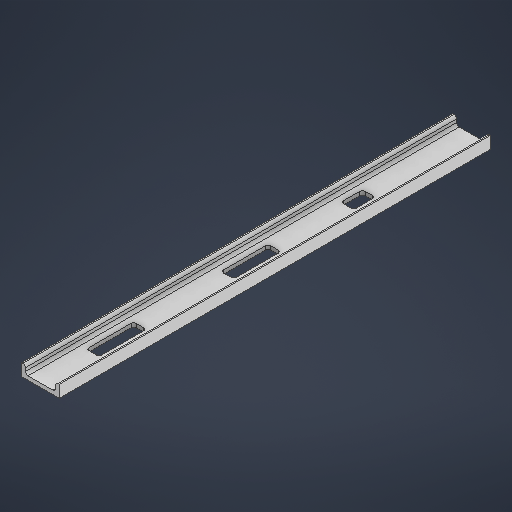
# Autodesk Inventor part: 2 часть направляшки 35
Saved by Autodesk Inventor 2025 (Build 290162000, 162)
## iProperties
Created: 2024-11-23
Part Number: 2 часть направляшки 35
Material: Типовые
Document SubType Name: Modeling
Designer: Phantom
Density: 1 g/cm^3
Appearance: По умолчанию
Author: Phantom
Autodesk Inventor part; units mm, degrees
ref_plane "YZ Plane" through (0, 0, 0) normal (1, 0, 0) x (0, 1, 0)
ref_plane "XZ Plane" through (0, 0, 0) normal (0, 1, 0) x (-1, 0, 0)
ref_plane "XY Plane" through (0, 0, 0) normal (0, 0, 1) x (1, 0, 0)
sketch "Эскиз1" plane through (0, 0, 0) normal (0, 0, 1) x (1, 0, 0)
  line L0 (0, 0) -> (34.5, 0)
  line L1 (34.5, 0) -> (34.5, 9.5)
  line L2 (34.5, 9.5) -> (0, 9.5)
  line L3 (0, 9.5) -> (0, 0)
  line L4 (3, 9.5) -> (3, 0)
  line L5 (31.5, 9.5) -> (31.5, 0)
  line L6 (3, 3) -> (31.5, 3)
  dimension "d0" = 34.5
  dimension "d1" = 9.5
  dimension "d2" = 3
  dimension "d3" = 3
  dimension "d4" = 3
  constraints: 14 end point, 6 point on line, 4 perpendicular, 2 parallel, 1 horizontal
  measures "d0" distance of L2.end L1.end
  measures "d1" distance of L1.end L0.end
  measures "d2" distance between parallel lines of L3 L4
  measures "d3" distance between parallel lines of L5 L1
  measures "d4" distance between parallel lines of L0 L6
extrude "Выдавливание1" add sketch "Эскиз1" along normal blind 388 contours L3 L2 L4 L0 | L4 L6 L5 L0 | L5 L2 L1 L0
sketch "Эскиз2" plane through (0, 0, 0) normal (0, -1, 0) x (1, 0, 0)
  line L0 (0, 0) -> (34.5, 0) projected
  line L1 (34.5, 0) -> (34.5, 388) projected
  line L2 (0, 388) -> (34.5, 388) projected
  line L3 (0, 0) -> (0, 388) projected
  line L4 (17.25, 388) -> (17.25, 0)
  line L5 (22.25, 310) -> (12.25, 310)
  line L6 (12.25, 310) -> (12.25, 347)
  line L7 (12.25, 347) -> (22.25, 347)
  line L8 (22.25, 347) -> (22.25, 310)
  line L9 (22.25, 310) -> (12.25, 347) construction
  line L10 (12.25, 310) -> (22.25, 347) construction
  line L11 (12.25, 204.5) -> (22.25, 204.5)
  line L12 (22.25, 204.5) -> (22.25, 241.5)
  line L13 (22.25, 241.5) -> (12.25, 241.5)
  line L14 (12.25, 241.5) -> (12.25, 204.5)
  line L15 (12.25, 204.5) -> (22.25, 241.5) construction
  line L16 (22.25, 204.5) -> (12.25, 241.5) construction
  line L17 (22.25, 130.5) -> (12.25, 130.5)
  line L18 (12.25, 130.5) -> (12.25, 147.5)
  line L19 (12.25, 147.5) -> (22.25, 147.5)
  line L20 (22.25, 147.5) -> (22.25, 130.5)
  line L21 (22.25, 130.5) -> (12.25, 147.5) construction
  line L22 (12.25, 130.5) -> (22.25, 147.5) construction
  point P0 (17.25, 328.5)
  point P1 (17.25, 223)
  point P2 (17.25, 139)
  dimension "d8" = 10
  dimension "d9" = 37
  dimension "d10" = 41
  dimension "d11" = 10
  dimension "d12" = 37
  dimension "d13" = 68.5
  dimension "d14" = 10
  dimension "d15" = 17
  dimension "d16" = 57
  constraints: 38 end point, 8 midpoint, 6 parallel, 3 horizontal, 3 perpendicular, 3 point on line
  measures "d8" distance of L6.end L7.end
  measures "d9" distance of L5.end L6.end
  measures "d10" distance between parallel lines of L7 L2
  measures "d11" distance of L13.end L12.end
  measures "d12" distance of L12.end L11.end
  measures "d13" distance between parallel lines of L13 L5
  measures "d14" distance of L18.end L19.end
  measures "d15" distance of L17.end L18.end
  measures "d16" distance between parallel lines of L19 L11
extrude "Выдавливание2" cut sketch "Эскиз2" against normal blind 295 contours L17 L18 L19 L4 | L4 L19 L20 L17 | L7 L8 L5 L4 | L4 L5 L6 L7 | L11 L14 L13 L4 | L4 L13 L12 L11
fillet "Сопряжение2" radius 2 12 edges at (12.25, 1.5, 241.5) (12.25, 1.5, 204.5) (22.25, 1.5, 204.5) (22.25, 1.5, 241.5) (22.25, 1.5, 147.5) (22.25, 1.5, 130.5) (12.25, 1.5, 147.5) (12.25, 1.5, 130.5) (12.25, 1.5, 310) (12.25, 1.5, 347) (22.25, 1.5, 347) (22.25, 1.5, 310)
sketch "Эскиз3" plane through (0, 0, 388) normal (0, 0, 1) x (1, 0, 0)
  line L0 (3, 3) -> (3, 9.5) projected
  line L1 (3, 9.5) -> (5.5, 9.5)
  line L2 (5.5, 9.5) -> (5.5, 0)
  line L3 (5.5, 0) -> (3, 0)
  line L4 (3, 0) -> (3, 9.5)
  line L5 (31.5, 9.5) -> (31.5, 3) projected
  line L6 (31.5, 9.5) -> (29, 9.5)
  line L7 (29, 9.5) -> (29, 0)
  line L8 (29, 0) -> (31.5, 0)
  line L9 (31.5, 0) -> (31.5, 9.5)
  point P0 (0, 0)
  dimension "d20" = 2.5
  dimension "d21" = 2.5
  constraints: 16 end point, 4 parallel, 2 horizontal, 2 perpendicular, 1 point on line
  measures "d20" distance of L2.end L3.end
  measures "d21" distance of L8.end L7.end
extrude "Выдавливание3" add sketch "Эскиз3" against normal up to surface (388 mm away)
sketch "Эскиз4" plane through (0, 0, 0) normal (0, 0, -1) x (-1, 0, 0)
  line L0 (-34.5, 9.5) -> (-29, 9.5) projected
  line L1 (0, 0) -> (-34.5, 0) projected
  line L2 (-34.5, 9.5) -> (-32, 9.5)
  line L3 (-32, 9.5) -> (-32, 0)
  line L4 (-32, 0) -> (-34.5, 0)
  line L5 (-34.5, 0) -> (-34.5, 9.5)
  line L6 (0, 9.5) -> (0, 0) projected
  line L7 (0, 9.5) -> (-2.5, 9.5)
  line L8 (-2.5, 9.5) -> (-2.5, 0)
  line L9 (-2.5, 0) -> (0, 0)
  line L10 (0, 0) -> (0, 9.5)
  dimension "d24" = 2.5
  dimension "d25" = 2.5
  constraints: 16 end point, 4 parallel, 2 horizontal, 2 perpendicular, 2 point on line
  measures "d24" distance of L3.end L4.end
  measures "d25" distance of L9.end L8.end
extrude "Выдавливание4" cut sketch "Эскиз4" against normal through all
fillet "Сопряжение3" radius 2 4 edges at (5.5, 3, 194) (29, 3, 194) (29, 9.5, 194) (5.5, 9.5, 194)
sketch "Эскиз5" plane through (0, 0, 0) normal (0, 0, -1) x (-1, 0, 0)
  line L0 (52, 100) -> (-112, 100)
  line L1 (-112, 100) -> (-112, -123)
  line L2 (-112, -123) -> (52, -123)
  line L3 (52, -123) -> (52, 100)
  point P0 (0, 0)
  constraints: 8 end point, 2 parallel, 1 horizontal, 1 perpendicular
extrude "Выдавливание5" cut sketch "Эскиз5" against normal blind 50
